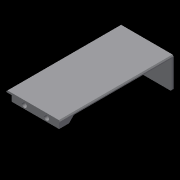
# Autodesk Inventor part: carcasainferior
Saved by Autodesk Inventor 2016 (Build 200138000, 138)
## iProperties
Created: 2017-08-15
Part Number: carcasainferior
Material: Generic
Document SubType Name: Modeling
Designer: ludwi
Density: 1 g/cm^3
Appearance: Default
Author: ludwi
Autodesk Inventor part; units mm, degrees
ref_plane "YZ Plane" through (0, 0, 0) normal (1, 0, 0) x (0, 1, 0)
ref_plane "XZ Plane" through (0, 0, 0) normal (0, 1, 0) x (-1, 0, 0)
ref_plane "XY Plane" through (0, 0, 0) normal (0, 0, 1) x (1, 0, 0)
sketch "Sketch1" plane through (0, 0, 0) normal (0, 0, 1) x (1, 0, 0)
  line L0 (0, 44.4) -> (0, 0) construction
  line L1 (0, 44.4) -> (-0.8, 44.4) construction
  line L2 (-0.8, 44.4) -> (-0.8, -0.8) construction
  line L3 (20.8, -0.8) -> (-0.8, -0.8) construction
  line L4 (20.8, 44.4) -> (20.8, -0.8) construction
  line L5 (20, 44.4) -> (20.8, 44.4) construction
  line L6 (20, 44.4) -> (20, 0) construction
  line L7 (20, 0) -> (0, 0) construction
  line L8 (-0.8, -0.8) -> (20.8, -0.8)
  line L9 (20.8, -0.8) -> (20.8, 44.4)
  line L10 (20.8, 44.4) -> (-0.8, 44.4)
  line L11 (-0.8, 44.4) -> (-0.8, -0.8)
  constraints: 8 end point, 2 parallel, 1 horizontal, 1 perpendicular
extrude "Extrusion1" add sketch "Sketch1" along normal blind 0.8
sketch "Sketch2" plane through (-0.8, 44.4, 0) normal (0, 1, 0) x (1, 0, 0)
  line L0 (7.1248, 6.15) -> (6.7248, 5.75) construction
  line L1 (7.1248, 10.1) -> (7.1248, 6.15) construction
  line L2 (7.5248, 10.5) -> (7.1248, 10.1) construction
  line L3 (7.5248, 10.5) -> (20.4, 10.5) construction
  line L4 (20.8, 10.1) -> (20.4, 10.5) construction
  line L5 (20.8, 10.1) -> (20.8, 0) construction
  line L6 (20.8, 0) -> (21.6, 0) construction
  line L7 (21.6, 11.1) -> (21.6, 0) construction
  line L8 (21.2, 11.5) -> (21.6, 11.1) construction
  line L9 (21.2, 11.5) -> (0.4, 11.5) construction
  line L10 (0, 11.1) -> (0.4, 11.5) construction
  line L11 (0, 0) -> (0, 11.1) construction
  line L12 (0.8, 0) -> (0, 0) construction
  line L13 (0.8, 0) -> (0.8, 5.35) construction
  line L14 (1.2, 5.75) -> (0.8, 5.35) construction
  line L15 (6.7248, 5.75) -> (1.2, 5.75) construction
  circle A0 centre (4.2195, 7.1194) radius 1 construction
  line L16 (21.6, -0.8) -> (0, -0.8) construction
  line L17 (0, -0.8) -> (21.6, -0.8) projected
  line L18 (0, -0.8) -> (21.6, -0.8)
  line L19 (21.6, -0.8) -> (21.6, 11.5)
  line L20 (21.6, 11.5) -> (0, 11.5)
  line L21 (0, 11.5) -> (0, -0.8)
  circle A1 centre (4.2195, 7.1194) radius 1.2
  line L22 (14.4, 3.4) -> (14.4, 2.2) construction
  line L23 (13.4, 1.2) -> (14.4, 2.2) construction
  line L24 (13.4, 1.2) -> (8.2, 1.2) construction
  line L25 (7.2, 2.2) -> (8.2, 1.2) construction
  line L26 (7.2, 2.2) -> (7.2, 3.4) construction
  line L27 (7.2, 3.4) -> (14.4, 3.4) construction
  line L28 (7.8, 8.5) -> (7.8, 5.5) construction
  line L29 (7.8, 5.5) -> (0.8, 5.5) construction
  line L30 (0.8, 0) -> (0.8, 5.5) construction
  line L31 (0.8, 0) -> (20.8, 0) construction
  line L32 (20.8, 0) -> (20.8, 8.5) construction
  line L33 (20.8, 8.5) -> (7.8, 8.5) construction
  line L34 (14.6, 3.6) -> (14.6, 2.1172)
  line L35 (14.6, 2.1172) -> (13.4828, 1)
  line L36 (13.4828, 1) -> (8.1172, 1)
  line L37 (8.1172, 1) -> (7, 2.1172)
  line L38 (7, 2.1172) -> (7, 3.6)
  line L39 (7, 3.6) -> (14.6, 3.6)
  dimension "d18" = 0.2
  dimension "d34" = 0.2
  constraints: 20 end point, 2 parallel, 1 centre point, 1 horizontal, 1 perpendicular, 1 point on line, 1 vertical alignment, 5 other
  measures "d18" radial gap between concentric circles of A1 A0
  measures "d34" distance between parallel lines of L27 L39
extrude "Extrusion2" add sketch "Sketch2" along normal blind 0.8
sketch "Sketch3" plane through (0, 0, 0) normal (0, 0, -1) x (-1, 0, 0)
  line L0 (-20, 0) -> (0, 0) construction
  line L1 (-20, 44.4) -> (-20, 0) construction
  line L2 (0, 44.4) -> (0, 0) construction
  line L3 (-20, 11) -> (-20, 0) construction
  line L4 (0, 11) -> (-20, 11) construction
  line L5 (0, 0) -> (0, 11) construction
  line L6 (-20, 0) -> (0, 0) construction
  line L7 (-19.6, 0.1) -> (-0.4, 0.1)
  line L8 (-0.4, 0.1) -> (-0.4, 4.1)
  line L9 (-0.4, 4.1) -> (-19.6, 4.1)
  line L10 (-19.6, 4.1) -> (-19.6, 0.1)
  dimension "d6" = 4
  dimension "d7" = 0.4
  dimension "d8" = 0.4
  dimension "d9" = 0.1
  constraints: 8 end point, 2 parallel, 1 horizontal, 1 perpendicular
  measures "d6" distance of L9.end L7.start
  measures "d7" distance between parallel lines of L1 L10
  measures "d8" distance between parallel lines of L2 L8
  measures "d9" distance between parallel lines of L0 L7
extrude "Extrusion3" add sketch "Sketch3" along normal blind 3.2
chamfer "Chamfer4" distance 3.2 angle 45 1 edges at (10, 4.1, 0)
sketch "Sketch5" plane through (0.4, 0.1, 0) normal (0, -1, 0) x (1, 0, 0)
  circle A0 centre (14.1, -1.75) radius 1.1 projected
  circle A1 centre (5.1, -1.75) radius 1.1 projected
  circle A2 centre (14.1, -1.75) radius 1
  circle A3 centre (5.1, -1.75) radius 1
  point P0 (-0.4, 0)
  dimension "d33" = 2
  constraints: 2 centre point, 2 coincident, 1 equal radius
  measures "d33" diameter of A2
extrude "Extrusion5" cut sketch "Sketch5" against normal blind 16.45 contours A2 | A3
chamfer "Chamfer5" distance 0.4 angle 45 11 edges at (-0.8, 22.2, 0.8) (20.8, 22.2, 0.8) (-0.8, 44.8, -11.5) (20.8, 44.8, -11.5) (2.2195, 45.2, -7.1194) (10, 45.2, -3.6) (6.2, 45.2, -2.8586) (6.7586, 45.2, -1.5586) (10, 45.2, -1) (13.2414, 45.2, -1.5586) (13.8, 45.2, -2.8586)
body "Solid1"
